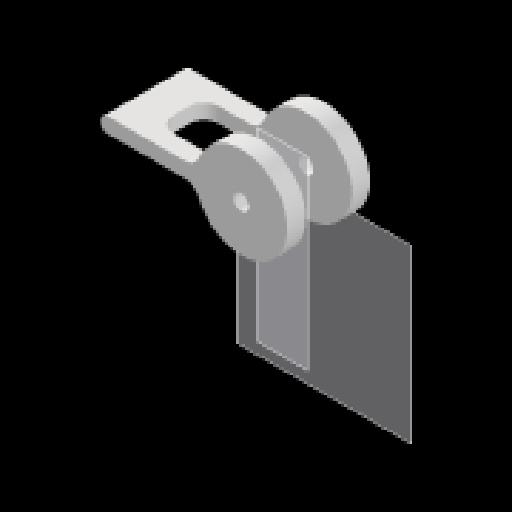
# Autodesk Inventor part: odomHousing
Saved by Autodesk Inventor 2024.1 (Build 281209000, 209)
## iProperties
Created: 2025-05-24
Part Number: odomHousing
Material: Generic
Document SubType Name: Modeling
Designer: Teddy
Density: 1 g/cm^3
Appearance: Default
Author: Teddy
Autodesk Inventor part; units mm, degrees
ref_plane "YZ Plane" through (0, 0, 0) normal (1, 0, 0) x (0, 1, 0)
ref_plane "XZ Plane" through (0, 0, 0) normal (0, 1, 0) x (-1, 0, 0)
ref_plane "XY Plane" through (0, 0, 0) normal (0, 0, 1) x (1, 0, 0)
ref_plane "Work Plane1" through (0, 0, 0) normal (0, 0, 1) x (1, 0, 0)
sketch "Sketch1" plane through (0, 0, 0) normal (0, 0, 1) x (1, 0, 0)
  circle A0 centre (0, 0) radius 3.175 projected
  circle A1 centre (0, 50.8) radius 19.05
  line L0 (0, 50.8) -> (-55.2684, 50.8) construction
  line L1 (0, 47.625) -> (-55.2684, 47.625)
  line L2 (-55.2684, 53.975) -> (0, 53.975)
  arc A2 (0, 47.625) -> (0, 53.975) centre (0, 50.8) ccw
  arc A3 (-55.2684, 53.975) -> (-55.2684, 47.625) centre (-55.2684, 50.8) ccw
  circle A4 centre (0, 50.8) radius 3.175
  circle A5 centre (0, 76.2) radius 2.286
  circle A6 centre (0, 76.2) radius 6.35
  line L3 (-5.4993, 79.375) -> (-16.4978, 60.325)
  line L4 (5.4993, 79.375) -> (16.4978, 60.325)
  point P0 (0, 25.4)
  point P1 (-27.6342, 50.8)
  point P2 (-18.7836, 47.625)
  point P3 (-18.7836, 53.975)
  dimension "d6" = 38.1
  dimension "d8" = 4.572
  dimension "d9" = 25.4
  constraints: 12 end point, 9 tangent, 8 point on circle, 6 centre point, 2 coincident, 1 horizontal, 1 midpoint, 1 parallel
  measures "d6" diameter of A1
  measures "d8" diameter of A5
  measures "d9" distance of L0.start A5.centre
extrude "Extrusion1" add sketch "Sketch1" along normal blind 34.29 contours A1 L1 A2 L2 | A1 A6 L4 | L1 A3 L2 A1 | A1 L2 A4 L1 | A1 L3 A6 | A6
ref_plane "Work Plane2" through (0, 0, 17.145) normal (0, 0, 1) x (1, 0, 0)
sketch "Sketch2" plane through (0, 0, 17.145) normal (0, 0, 1) x (1, 0, 0)
  arc A0 (-16.4978, 60.325) -> (-18.7836, 53.975) centre (0, 50.8) ccw projected
  line L0 (0, 0) -> (0, 50.8) construction
  line L1 (-9.525, 0) -> (-9.525, 50.8)
  line L2 (9.525, 50.8) -> (9.525, 0)
  arc A1 (9.525, 50.8) -> (-9.525, 50.8) centre (0, 50.8) ccw
  line L3 (-55.2684, 47.625) -> (-18.7836, 47.625) projected
  arc A2 (-55.2684, 53.975) -> (-55.2684, 47.625) centre (-55.2684, 50.8) ccw projected
  line L4 (-18.7836, 53.975) -> (-55.2684, 53.975) projected
  circle A3 centre (0, 50.8) radius 19.05
  line L5 (-55.2684, 47.625) -> (-18.7836, 47.625) projected
  line L6 (-42.2273, 47.625) -> (-42.2273, 53.975)
  line L7 (-5.4993, 79.375) -> (-16.4978, 60.325) projected
  arc A4 (5.4993, 79.375) -> (-5.4993, 79.375) centre (0, 76.2) ccw projected
  line L8 (16.4978, 60.325) -> (5.4993, 79.375) projected
  arc A5 (-18.7836, 47.625) -> (16.4978, 60.325) centre (0, 50.8) ccw projected
  point P0 (9.525, 34.3022)
  point P1 (-9.525, 34.3022)
  point P2 (9.525, 34.3022)
  point P3 (-9.525, 34.3022)
  point P4 (-16.4978, 60.325)
  constraints: 10 end point, 2 centre point, 2 point on circle, 2 point on line, 2 tangent, 1 concentric, 1 parallel, 1 perpendicular, 1 vertical
extrude "Extrusion2" cut sketch "Sketch2" along normal mid plane 19.05 contours A3 L2 A1 L1 A0 | L7 A4 L8 A3 | A3 L3 L6 L4 | L1 A1 L2 A3
fillet "Fillet1" radius 6.35 6 edges at (-42.2273, 50.8, 7.62) (-42.2273, 50.8, 26.67) (-18.7836, 53.975, 30.48) (-18.7836, 47.625, 30.48) (-18.7836, 53.975, 3.81) (-18.7836, 47.625, 3.81)
body "Solid1"
